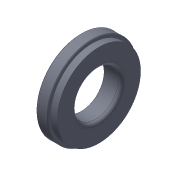
# Autodesk Inventor part: NA-45-h-Crown-217
Saved by Autodesk Inventor 2020.2 (Build 242310000, 310)
## iProperties
Created: 2020-09-21
Part Number: NA-45-h-Crown-217
Material: 19 436.4
Document SubType Name: Modelování
Designer: Jurek
Mass: 436.922 g
Surface Area: 131.089 cm^2
Volume: 55.6589 cm^3
Density: 7.85 g/cm^3
Appearance: RAL 7040 Window Grey(1)
Description: NAVÁDĚCÍ KROUŽEK
Sheet Metal Rule: Výchozí
User Status: Rozpracováno
Category: B
Hmotnost (kg): 0,43
Rozmer_A: 80
Rozmer_B: 0
Rozmer_C: 0,5
Rozmer_D: 16
Rada vyrobku: 4100
Prumer nadobky: 45
Cislo artiklu: 4451101341
C. variantniho vykresu: NA-45-h-Crown-217
Jednotka: ks
Cisty rozmer: =Ø<Rozmer_A> - <Rozmer_D>
Predpona: Ø
Stroj na lince: Stahovací lis
RAZ Poznamka 1: ISO 2768-mH
RAZ Poznamka 2: NEOZNAČENÉ HRANY OJEHLIT
RAZ Poznamka 3: KALIT NA 58 - 60 HRc
DXF: Ne
QAD_code: M
Rizeni davek: L
Author: Správce
Revision Number: 00
Autodesk Inventor part; units mm, degrees
ref_plane "YZ Plane" through (0, 0, 0) normal (1, 0, 0) x (0, 1, 0)
ref_plane "XZ Plane" through (0, 0, 0) normal (0, 1, 0) x (-1, 0, 0)
ref_plane "XY Plane" through (0, 0, 0) normal (0, 0, 1) x (1, 0, 0)
sketch "Náčrt1" plane through (0, 0, 0) normal (0, 0, 1) x (1, 0, 0)
  line L0 (0, 0) -> (18.405, 0)
  line L1 (0, 20.165) -> (0, 40)
  line L2 (0, 40) -> (10, 40)
  line L3 (10, 40) -> (10, 37.25)
  line L4 (10, 37.25) -> (16, 37.25)
  line L5 (16, 37.25) -> (16, 20.165)
  line L6 (16, 20.165) -> (0, 20.165)
  dimension "d0" = 80
  dimension "d1" = 40.33
  dimension "d2" = 74.5
  dimension "d3" = 16
  dimension "d4" = 10
  constraints: 14 end point, 4 parallel, 2 perpendicular, 1 horizontal, 1 point on line
  measures "d0" diameter of L2 L0
  measures "d1" diameter of L6 L0
  measures "d2" diameter of L4 L0
  measures "d3" distance between parallel lines of L1 L5
  measures "d4" distance between parallel lines of L3 L1
revolve "Rotace1" add sketch "Náčrt1" angle 360 about axis through (0, 0, 0) along (1, 0, 0)
fillet "Zaoblení1" radius 3 1 edges at (16, -20.165, 0)
fillet "Zaoblení2" radius 0.5 1 edges at (0, -20.165, 0)
chamfer "Zkosení1" distance 0.5 angle 45 2 edges at (0, -40, 0) (10, -40, 0)
equation "\"PoloměrOhybu\" = Tloušťka"
equation "\"ŠířkaVýštipu\" = Tloušťka"
equation "\"HloubkaVýštipu\" = 0.5 * Tloušťka"
equation "\"VelikostRohovéhoVýštipu\" = 4 * Tloušťka"
equation "\"MinimálníZbytek\" = 2 * Tloušťka"
equation "\"PřechodovýPoloměr\" = PoloměrOhybu"
equation "\"VelikostJacobihoPoloměru\" = Tloušťka"
equation "\"VelikostMezery\" = Tloušťka"
equation "\"Rozmer_B\" = 0"
equation "\"Rozmer_C\" = Tloušťka"
equation "\"Rozmer_D\" = d3"
equation "\"Tloušťka\" = 0.5"
